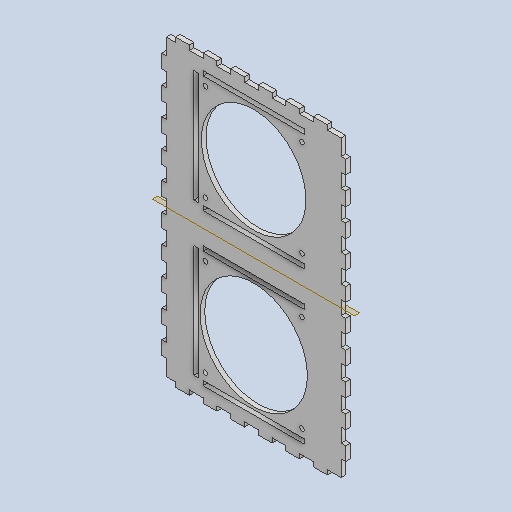
# Autodesk Inventor part: BackFrontPannel
Saved by Autodesk Inventor 2023 (Build 270158000, 158)
## iProperties
Created: 2022-09-19
Part Number: BackFrontPannel
Material: Generic
Document SubType Name: Modeling
Designer: Nathann
Density: 1 g/cm^3
Appearance: Default
Author: Nathann
Autodesk Inventor part; units mm, degrees
ref_plane "YZ Plane" through (0, 0, 0) normal (1, 0, 0) x (0, 1, 0)
ref_plane "XZ Plane" through (0, 0, 0) normal (0, 1, 0) x (-1, 0, 0)
ref_plane "XY Plane" through (0, 0, 0) normal (0, 0, 1) x (1, 0, 0)
sketch "Sketch1" plane through (0, 0, 0) normal (0, 0, 1) x (1, 0, 0)
  line L0 (0, 0) -> (200, 0)
  line L1 (200, 0) -> (200, -330)
  line L2 (200, -330) -> (0, -330)
  line L3 (0, -330) -> (0, 0)
  dimension "d0" = 200
  dimension "d1" = 330
  constraints: 8 end point, 2 parallel, 1 horizontal, 1 perpendicular
  measures "d0" distance of L0.start L0.end
  measures "d1" distance of L2.end L0.start
extrude "Extrusion1" add sketch "Sketch1" along normal blind 5
sketch "Sketch2" plane through (0, 0, 0) normal (0, 0, -1) x (-1, 0, 0)
  line L0 (0, 0) -> (-5, 0)
  line L1 (-5, 0) -> (-5, -22.5)
  line L2 (-5, -22.5) -> (0, -22.5)
  line L3 (0, -22.5) -> (0, 0)
  line L4 (-200, 0) -> (0, 0) projected
  line L5 (0, 0) -> (0, -330) projected
  line L6 (0, -37.5) -> (-5, -37.5)
  line L7 (-5, -37.5) -> (-5, -52.5)
  line L8 (-5, -52.5) -> (0, -52.5)
  line L9 (0, -52.5) -> (0, -37.5)
  line L10 (0, -30) -> (-5, -30)
  line L11 (0, -67.5) -> (-5, -67.5)
  line L12 (-5, -67.5) -> (-5, -82.5)
  line L13 (-5, -82.5) -> (0, -82.5)
  line L14 (0, -82.5) -> (0, -67.5)
  line L15 (0, -60) -> (-5, -60)
  line L16 (0, -97.5) -> (-5, -97.5)
  line L17 (-5, -97.5) -> (-5, -112.5)
  line L18 (-5, -112.5) -> (0, -112.5)
  line L19 (0, -112.5) -> (0, -97.5)
  line L20 (0, -90) -> (-5, -90)
  line L21 (0, -127.5) -> (-5, -127.5)
  line L22 (-5, -127.5) -> (-5, -142.5)
  line L23 (-5, -142.5) -> (0, -142.5)
  line L24 (0, -142.5) -> (0, -127.5)
  line L25 (0, -120) -> (-5, -120)
  line L26 (0, -157.5) -> (-5, -157.5)
  line L27 (-5, -157.5) -> (-5, -172.5)
  line L28 (-5, -172.5) -> (0, -172.5)
  line L29 (0, -172.5) -> (0, -157.5)
  line L30 (0, -150) -> (-5, -150)
  line L31 (0, -187.5) -> (-5, -187.5)
  line L32 (-5, -187.5) -> (-5, -202.5)
  line L33 (-5, -202.5) -> (0, -202.5)
  line L34 (0, -202.5) -> (0, -187.5)
  line L35 (0, -180) -> (-5, -180)
  line L36 (0, -217.5) -> (-5, -217.5)
  line L37 (-5, -217.5) -> (-5, -232.5)
  line L38 (-5, -232.5) -> (0, -232.5)
  line L39 (0, -232.5) -> (0, -217.5)
  line L40 (0, -210) -> (-5, -210)
  line L41 (0, -247.5) -> (-5, -247.5)
  line L42 (-5, -247.5) -> (-5, -262.5)
  line L43 (-5, -262.5) -> (0, -262.5)
  line L44 (0, -262.5) -> (0, -247.5)
  line L45 (0, -330) -> (-5, -330)
  line L46 (-5, -330) -> (-5, -307.5)
  line L47 (-5, -307.5) -> (0, -307.5)
  line L48 (0, -307.5) -> (0, -330)
  line L49 (-200, 0) -> (0, 0) projected
  line L50 (-100, 0) -> (-100, -60)
  line L51 (-200, 0) -> (-195, 0)
  line L52 (-195, 0) -> (-195, -22.5)
  line L53 (-195, -22.5) -> (-200, -22.5)
  line L54 (-200, -22.5) -> (-200, 0)
  line L55 (0, 0) -> (-200, 0)
  line L56 (-200, 0) -> (-200, -330)
  line L57 (-200, -37.5) -> (-195, -37.5)
  line L58 (-195, -37.5) -> (-195, -52.5)
  line L59 (-195, -52.5) -> (-200, -52.5)
  line L60 (-200, -52.5) -> (-200, -37.5)
  line L61 (-200, -30) -> (-195, -30)
  line L62 (-200, -67.5) -> (-195, -67.5)
  line L63 (-195, -67.5) -> (-195, -82.5)
  line L64 (-195, -82.5) -> (-200, -82.5)
  line L65 (-200, -82.5) -> (-200, -67.5)
  line L66 (-200, -60) -> (-195, -60)
  line L67 (-200, -97.5) -> (-195, -97.5)
  line L68 (-195, -97.5) -> (-195, -112.5)
  line L69 (-195, -112.5) -> (-200, -112.5)
  line L70 (-200, -112.5) -> (-200, -97.5)
  line L71 (-200, -90) -> (-195, -90)
  line L72 (-200, -127.5) -> (-195, -127.5)
  line L73 (-195, -127.5) -> (-195, -142.5)
  line L74 (-195, -142.5) -> (-200, -142.5)
  line L75 (-200, -142.5) -> (-200, -127.5)
  line L76 (-200, -120) -> (-195, -120)
  line L77 (-200, -157.5) -> (-195, -157.5)
  line L78 (-195, -157.5) -> (-195, -172.5)
  line L79 (-195, -172.5) -> (-200, -172.5)
  line L80 (-200, -172.5) -> (-200, -157.5)
  line L81 (-200, -150) -> (-195, -150)
  line L82 (-200, -187.5) -> (-195, -187.5)
  line L83 (-195, -187.5) -> (-195, -202.5)
  line L84 (-195, -202.5) -> (-200, -202.5)
  line L85 (-200, -202.5) -> (-200, -187.5)
  line L86 (-200, -180) -> (-195, -180)
  line L87 (-200, -217.5) -> (-195, -217.5)
  line L88 (-195, -217.5) -> (-195, -232.5)
  line L89 (-195, -232.5) -> (-200, -232.5)
  line L90 (-200, -232.5) -> (-200, -217.5)
  line L91 (-200, -210) -> (-195, -210)
  line L92 (-200, -247.5) -> (-195, -247.5)
  line L93 (-195, -247.5) -> (-195, -262.5)
  line L94 (-195, -262.5) -> (-200, -262.5)
  line L95 (-200, -262.5) -> (-200, -247.5)
  line L96 (-200, -330) -> (-195, -330)
  line L97 (-195, -330) -> (-195, -307.5)
  line L98 (-195, -307.5) -> (-200, -307.5)
  line L99 (-200, -307.5) -> (-200, -330)
  line L100 (0, 0) -> (-200, 0)
  line L101 (0, -240) -> (-5, -240)
  line L102 (0, -277.5) -> (-5, -277.5)
  line L103 (-5, -277.5) -> (-5, -292.5)
  line L104 (-5, -292.5) -> (0, -292.5)
  line L105 (0, -292.5) -> (0, -277.5)
  line L106 (-200, -277.5) -> (-195, -277.5)
  line L107 (-195, -277.5) -> (-195, -292.5)
  line L108 (-195, -292.5) -> (-200, -292.5)
  line L109 (-200, -292.5) -> (-200, -277.5)
  point P0 (-200, -307.5)
  point P1 (0, -307.5)
  point P2 (-200, -187.5)
  point P3 (-200, -202.5)
  point P4 (0, -262.5)
  point P5 (0, -232.5)
  point P6 (0, -202.5)
  point P7 (-200, -82.5)
  point P8 (0, -172.5)
  point P9 (-200, -157.5)
  point P10 (-200, -172.5)
  point P11 (0, -142.5)
  point P12 (-200, -142.5)
  point P13 (0, -112.5)
  point P14 (-200, -97.5)
  point P15 (-200, -112.5)
  point P16 (0, -82.5)
  point P17 (-200, -247.5)
  point P18 (-200, -262.5)
  point P19 (-200, -22.5)
  point P20 (-195, 0)
  point P21 (-200, -232.5)
  point P22 (0, -292.5)
  point P23 (-200, -277.5)
  point P24 (-200, -292.5)
  dimension "d4" = 0
  dimension "d5" = 5
  dimension "d6" = 0
  dimension "d7" = 22.5
  dimension "d8" = 5
  dimension "d9" = 15
  dimension "d10" = 15
  dimension "d13" = 30
  dimension "d18" = 22.5
  dimension "d19" = 5
  constraints: 212 end point, 60 symmetric about line, 48 vertical alignment, 30 parallel, 16 collinear, 3 horizontal, 3 perpendicular, 1 midpoint, 1 vertical, 6 other
  measures "d4" distance between parallel lines of L4 L0
  measures "d5" distance of L1.end L2.end
  measures "d6" horizontal extent of L3
  measures "d7" distance of L0.end L1.end
  measures "d8" distance of L6.start L6.end
  measures "d9" distance of L6.end L7.end
  measures "d10" distance between parallel lines of L6 L2
  measures "d13" distance of L0.start L10.start
  measures "d18" distance of L45.end L46.end
  measures "d19" distance of L46.end L47.end
extrude "Extrusion2" cut sketch "Sketch2" against normal mid plane 20
sketch "Sketch3" plane through (0, 0, 5) normal (0, 0, 1) x (1, 0, 0)
  circle A0 centre (47.5, -30) radius 2.5
  circle A1 centre (152.5, -30) radius 2.5
  circle A2 centre (47.5, -135) radius 2.5
  circle A3 centre (152.5, -135) radius 2.5
  circle A4 centre (47.5, -195) radius 2.5
  circle A5 centre (152.5, -195) radius 2.5
  circle A6 centre (47.5, -300) radius 2.5
  circle A7 centre (152.5, -300) radius 2.5
  line L0 (5, 0) -> (5, -22.5) projected
  line L1 (195, -22.5) -> (195, 0) projected
  line L2 (5, -330) -> (195, -330) projected
  line L3 (195, 0) -> (5, 0) projected
  circle A8 centre (100, -82.5) radius 56.9012
  circle A9 centre (100, -247.5) radius 58.271
  line L4 (195, -202.5) -> (195, -187.5) projected
  point P0 (0, 0)
  dimension "d22" = 5
  dimension "d23" = 5
  dimension "d24" = 5
  dimension "d25" = 5
  dimension "d26" = 5
  dimension "d27" = 5
  dimension "d28" = 5
  dimension "d29" = 5
  dimension "d30" = 105
  dimension "d31" = 105
  dimension "d32" = 105
  dimension "d33" = 42.5
  dimension "d34" = 190
  dimension "d35" = 105
  dimension "d36" = 105
  dimension "d37" = 105
  dimension "d39" = 42.5
  dimension "d40" = 30
  dimension "d41" = 105
  dimension "d47" = 95
  dimension "d48" = 95
  dimension "d51" = 30
  dimension "d52" = 52.5
  dimension "d53" = 52.5
  constraints: 10 centre point, 3 vertical alignment, 2 horizontal alignment
  measures "d22" diameter of A0
  measures "d23" diameter of A1
  measures "d24" diameter of A2
  measures "d25" diameter of A3
  measures "d26" diameter of A4
  measures "d27" diameter of A5
  measures "d28" diameter of A6
  measures "d29" diameter of A7
  measures "d30" distance of A1.centre A0.centre
  measures "d31" distance of A3.centre A2.centre
  measures "d32" distance of A2.centre A0.centre
  measures "d33" distance from line of L0 A0.centre
  measures "d34" distance between parallel lines of L1 L0
  measures "d35" distance of A5.centre A4.centre
  measures "d36" distance of A7.centre A6.centre
  measures "d37" distance of A6.centre A4.centre
  measures "d39" distance from line of L0 A4.centre
  measures "d40" distance from line of L3 A0.centre
  measures "d41" distance of A7.centre A5.centre
  measures "d47" distance from line of L4 A9.centre
  measures "d48" distance from line of L0 A8.centre
  measures "d51" distance from line of L2 A7.centre
  measures "d52" horizontal distance of A8.centre A1.centre
  measures "d53" horizontal distance of A5.centre A9.centre
extrude "Extrusion3" cut sketch "Sketch3" along normal mid plane 20
sketch "Sketch4" plane through (0, 0, 5) normal (0, 0, 1) x (1, 0, 0)
  line L0 (155, -16.5) -> (45, -16.5) projected
  line L1 (155, -21.5) -> (45, -21.5) projected
  line L2 (155, -21.5) -> (155, -16.5) projected
  line L3 (45, -16.5) -> (45, -21.5) projected
  line L4 (155, -148.5) -> (45, -148.5) projected
  line L5 (155, -143.5) -> (45, -143.5) projected
  line L6 (155, -148.5) -> (155, -143.5) projected
  line L7 (45, -143.5) -> (45, -148.5) projected
  line L8 (155, -181.5) -> (45, -181.5) projected
  line L9 (155, -186.5) -> (45, -186.5) projected
  line L10 (155, -186.5) -> (155, -181.5) projected
  line L11 (45, -181.5) -> (45, -186.5) projected
  line L12 (155, -313.5) -> (45, -313.5) projected
  line L13 (155, -308.5) -> (45, -308.5) projected
  line L14 (155, -313.5) -> (155, -308.5) projected
  line L15 (45, -308.5) -> (45, -313.5) projected
  point P0 (0, 0)
extrude "Extrusion4" cut sketch "Sketch4" against normal blind 10
sketch "Sketch5" plane through (0, 0, 5) normal (0, 0, 1) x (1, 0, 0)
  line L0 (35, -21.5) -> (35, -143.5) projected
  line L1 (40, -143.5) -> (40, -21.5) projected
  line L2 (40, -21.5) -> (35, -21.5) projected
  line L3 (35, -143.5) -> (40, -143.5) projected
  line L4 (35, -186.5) -> (35, -308.5) projected
  line L5 (40, -308.5) -> (40, -186.5) projected
  line L6 (40, -186.5) -> (35, -186.5) projected
  line L7 (35, -308.5) -> (40, -308.5) projected
  point P0 (0, 0)
extrude "Extrusion5" cut sketch "Sketch5" against normal blind 10
sketch "Sketch6" plane through (0, 0, 5) normal (0, 0, 1) x (1, 0, 0)
  line L0 (0, 0) -> (15, 0)
  line L1 (15, 0) -> (15, -5)
  line L2 (15, -5) -> (0, -5)
  line L3 (0, -5) -> (0, 0)
  line L4 (30, 0) -> (45, 0)
  line L5 (45, 0) -> (45, -5)
  line L6 (45, -5) -> (30, -5)
  line L7 (30, -5) -> (30, 0)
  line L8 (60, 0) -> (75, 0)
  line L9 (75, 0) -> (75, -5)
  line L10 (75, -5) -> (60, -5)
  line L11 (60, -5) -> (60, 0)
  line L12 (90, 0) -> (105, 0)
  line L13 (105, 0) -> (105, -5)
  line L14 (105, -5) -> (90, -5)
  line L15 (90, -5) -> (90, 0)
  line L16 (120, 0) -> (135, 0)
  line L17 (135, 0) -> (135, -5)
  line L18 (135, -5) -> (120, -5)
  line L19 (120, -5) -> (120, 0)
  line L20 (150, 0) -> (165, 0)
  line L21 (165, 0) -> (165, -5)
  line L22 (165, -5) -> (150, -5)
  line L23 (150, -5) -> (150, 0)
  line L24 (180, 0) -> (195, 0)
  line L25 (195, 0) -> (195, -5)
  line L26 (195, -5) -> (180, -5)
  line L27 (180, -5) -> (180, 0)
  point P0 (195, 0)
  dimension "d58" = 5
  dimension "d59" = 15
  dimension "d62" = 30
  constraints: 56 end point, 2 horizontal, 2 parallel, 1 collinear, 1 perpendicular, 47 other
  measures "d58" distance of L2.end L0.start
  measures "d59" distance of L1.end L2.end
  measures "d62" distance of L1.end L5.end
extrude "Extrusion6" cut sketch "Sketch6" against normal blind 10
ref_plane "Work Plane1" through (165, -165, 0) normal (0, 1, 0) x (1, 0, 0)
mirror "Mirror1" about plane through (165, -165, 0) normal (0, 1, 0) of "Extrusion6"
equation "\"d2\" = WoodWidth"
equation "\"d5\" = WoodWidth - LaserWith"
equation "\"d8\" = d5"
equation "\"d18\" = d7"
equation "\"d19\" = d5"
equation "\"d20\" = 4 * WoodWidth"
equation "\"d33\" = -0.5 * d30 + 0.5 * d34"
equation "\"d39\" = d33"
equation "\"d40\" = d38"
equation "\"d47\" = d48"
equation "\"d48\" = 0.5 * d34"
equation "\"d51\" = d40"
equation "\"d52\" = 0.5 * d32"
equation "\"d53\" = d52"
equation "\"d42\" = 4 * WoodWidth"
equation "\"WoodWidth\" = 5"
equation "\"LaserWith\" = 0"
equation "\"d38\" = 30"
body "Solid1"
